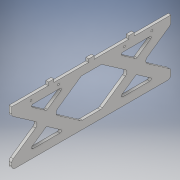
# Autodesk Inventor part: landingGear
Saved by Autodesk Inventor 2018 (Build 220112000, 112)
## iProperties
Created: 2020-01-24
Part Number: landingGear
Material: Generic
Document SubType Name: Modeling
Designer: anirudh.bali
Density: 1 g/cm^3
Appearance: Default
Author: anirudh.bali
Autodesk Inventor part; units mm, degrees
ref_plane "YZ Plane" through (0, 0, 0) normal (1, 0, 0) x (0, 1, 0)
ref_plane "XZ Plane" through (0, 0, 0) normal (0, 1, 0) x (-1, 0, 0)
ref_plane "XY Plane" through (0, 0, 0) normal (0, 0, 1) x (1, 0, 0)
sketch "Sketch1" plane through (0, 0, 0) normal (1, 0, 0) x (0, 1, 0)
  line L0 (132.588, -294.2082) -> (132.6134, -294.2082)
  line L1 (127, -262.509) -> (127, -252.349)
  line L2 (127, -190.2714) -> (127, -180.1114)
  line L3 (132.588, -67.818) -> (127, -67.818)
  line L4 (132.588, -77.978) -> (127, -77.978)
  line L5 (132.588, -142.0368) -> (127, -142.0368)
  line L6 (132.588, -152.1968) -> (127, -152.1968)
  line L7 (132.588, -216.2302) -> (127, -216.2302)
  line L8 (132.588, -226.3902) -> (127, -226.3902)
  line L9 (132.588, -216.2302) -> (132.588, -226.3902)
  line L10 (132.588, -67.818) -> (132.588, -77.978)
  line L11 (132.588, -142.0368) -> (132.588, -152.1968)
  line L12 (127, 0) -> (127, -67.818)
  line L13 (127, -77.978) -> (127, -142.0368)
  line L14 (127, -152.1968) -> (127, -216.2302)
  line L15 (127, -226.3902) -> (127, -294.2082)
  line L16 (25.4, 0) -> (25.4, -294.2082)
  line L17 (127, 0) -> (112, 0)
  line L18 (25.4, 0) -> (40.4, 0)
  line L19 (127, -294.2082) -> (112, -294.2082)
  line L20 (40.4, -294.2082) -> (25.4, -294.2082)
  line L21 (127, 0) -> (112, 0)
  line L22 (40.4, 0) -> (25.4, 0)
  line L23 (112, 0) -> (76.2, -51.435)
  line L24 (40.4, 0) -> (76.2, -51.435)
  line L25 (40.4, -128.27) -> (76.2, -76.835)
  line L26 (76.2, -76.835) -> (112, -128.27)
  line L27 (88.9, -64.135) -> (112, -30.9465)
  line L28 (88.9, -64.135) -> (112, -97.3235)
  line L29 (63.5, -64.135) -> (40.4, -30.9465)
  line L30 (63.5, -64.135) -> (40.4, -97.3235)
  line L31 (112, -30.9465) -> (112, -97.3235)
  line L32 (40.4, -97.3235) -> (40.4, -30.9465)
  line L33 (112, -294.2082) -> (76.2, -242.7732)
  line L34 (40.4, -294.2082) -> (76.2, -242.7732)
  line L35 (40.4, -165.9382) -> (76.2, -217.3732)
  line L36 (76.2, -217.3732) -> (112, -165.9382)
  line L37 (88.9, -230.0732) -> (112, -263.2617)
  line L38 (88.9, -230.0732) -> (112, -196.8847)
  line L39 (63.5, -230.0732) -> (40.4, -263.2617)
  line L40 (63.5, -230.0732) -> (40.4, -196.8847)
  line L41 (112, -263.2617) -> (112, -196.8847)
  line L42 (40.4, -196.8847) -> (40.4, -263.2617)
  line L43 (112, -128.27) -> (112, -165.9382)
  line L44 (112, -196.8847) -> (112, -263.2617)
  line L45 (40.4, -263.2617) -> (40.4, -196.8847)
  line L46 (40.4, -165.9382) -> (40.4, -128.27)
  point P0 (0, 0)
  dimension "d49" = 15
  constraints: 94 end point, 26 perpendicular, 13 parallel, 7 vertical, 4 horizontal, 4 point on line
  measures "d49" distance of L18.end L16.start
extrude "Extrusion3" add sketch "Sketch1" along normal blind 5.08
fillet "Fillet7" radius 6.35 12 edges at (2.54, 112, 0) (2.54, 76.2, -51.435) (2.54, 40.4, 0) (2.54, 76.2, -76.835) (2.54, 112, -128.27) (2.54, 40.4, -128.27) (2.54, 40.4, -165.9382) (2.54, 112, -165.9382) (2.54, 76.2, -217.3732) (2.54, 76.2, -242.7732) (2.54, 112, -294.2082) (2.54, 40.4, -294.2082)
fillet "Fillet8" radius 2.54 12 edges at (2.54, 112, -30.9465) (2.54, 88.9, -64.135) (2.54, 112, -97.3235) (2.54, 40.4, -30.9465) (2.54, 63.5, -64.135) (2.54, 40.4, -97.3235) (2.54, 112, -196.8847) (2.54, 88.9, -230.0732) (2.54, 112, -263.2617) (2.54, 63.5, -230.0732) (2.54, 40.4, -263.2617) (2.54, 40.4, -196.8847)
fillet "Fillet9" radius 6.35 2 edges at (2.54, 25.4, -294.2082) (2.54, 25.4, 0)
sketch "Sketch3" plane through (5.08, 0, 0) normal (1, 0, 0) x (0, 0, -1)
  line L0 (39.042, 112) -> (89.228, 112) projected
  circle A0 centre (35.3568, 119.5) radius 1.75
  circle A1 centre (86.1568, 119.5) radius 1.75
  line L1 (294.2082, 115.317) -> (294.2082, 127) projected
  circle A2 centre (258.8514, 119.5) radius 1.75
  circle A3 centre (208.0514, 119.5) radius 1.75
  point P0 (0, 0)
  point P1 (0, 127)
  dimension "d97" = 3.5
  dimension "d98" = 3.5
  constraints: 4 centre point
  measures "d97" diameter of A0
  measures "d98" diameter of A1
extrude "Extrusion5" cut sketch "Sketch3" against normal blind 25.4
body "Solid3"
